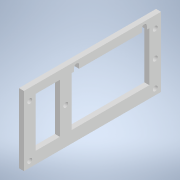
# Autodesk Inventor part: Soporte_PCB
Saved by Autodesk Inventor 2020.1 (Build 241239000, 239)
## iProperties
Created: 2019-12-12
Part Number: Soporte_PCB
Material: Generic
Document SubType Name: Modeling
Designer: Daniel
Density: 1 g/cm^3
Appearance: Default
Author: Daniel
Autodesk Inventor part; units mm, degrees
ref_plane "YZ Plane" through (0, 0, 0) normal (1, 0, 0) x (0, 1, 0)
ref_plane "XZ Plane" through (0, 0, 0) normal (0, 1, 0) x (-1, 0, 0)
ref_plane "XY Plane" through (0, 0, 0) normal (0, 0, 1) x (1, 0, 0)
sketch "Sketch1" plane through (0, 0, 0) normal (1, 0, 0) x (0, 1, 0)
  line L0 (-15.5, 37.5) -> (15.5, 37.5) construction
  line L1 (15.5, 37.5) -> (15.5, -37.5) construction
  line L2 (15.5, -37.5) -> (-15.5, -37.5) construction
  line L3 (-15.5, -37.5) -> (-15.5, 37.5) construction
  line L4 (-15.5, 37.5) -> (15.5, -37.5) construction
  line L5 (15.5, 37.5) -> (-15.5, -37.5) construction
  line L6 (-19, 41) -> (22.5, 41)
  line L7 (22.5, 41) -> (22.5, -41)
  line L8 (22.5, -41) -> (-19, -41)
  line L9 (-19, -41) -> (-19, 41)
  line L10 (-19, 41) -> (22.5, -41) construction
  line L11 (22.5, 41) -> (-19, -41) construction
  line L12 (-12, 34) -> (17.5, 34)
  line L13 (17.5, 34) -> (17.5, -34)
  line L14 (17.5, -34) -> (-12, -34)
  line L15 (-12, -34) -> (-12, 34)
  line L16 (-12, 34) -> (17.5, -34) construction
  line L17 (17.5, 34) -> (-12, -34) construction
  line L18 (-46.909, 0) -> (32.0039, 0) construction
  arc A0 (19.5, -32.5) -> (19.5, -29.5) centre (19.5, -31) ccw
  line L19 (19.5, -32.5) -> (17.5, -32.5)
  line L20 (19.5, -29.5) -> (17.5, -29.5)
  line L21 (19.5, -31) -> (19.5, -32.5) construction
  line L22 (19.5, -31) -> (19.5, -29.5) construction
  arc A1 (19.5, 8) -> (19.5, 11) centre (19.5, 9.5) ccw
  line L23 (19.5, 8) -> (17.5, 8)
  line L24 (19.5, 11) -> (17.5, 11)
  line L25 (19.5, 9.5) -> (19.5, -31) construction
  line L26 (22.5, -10.75) -> (19.5, -10.75) construction
  line L27 (17.5, 12.5) -> (-12, 12.5)
  line L28 (17.5, 19.5) -> (-12, 19.5)
  line L29 (17.5, 16) -> (-12, 16) construction
  point P0 (0, 0)
  point P1 (0, 0)
  point P2 (2.75, 0)
  point P3 (1.75, 0)
  point P4 (0, -37.5)
  point P5 (2.75, 16)
  dimension "d0" = 31
  dimension "d1" = 75
  dimension "d3" = 82
  dimension "d5" = 68
  dimension "d6" = 5
  dimension "d7" = 3.5
  dimension "d8" = 3.5
  dimension "d10" = 17.5
  dimension "d11" = 3
  dimension "d12" = 6.5
  dimension "d13" = 4
  dimension "d16" = 40.5
  dimension "d21" = 7
  dimension "d22" = 3.5
  constraints: 60 end point, 9 midpoint, 8 parallel, 8 point on line, 6 horizontal, 5 perpendicular, 4 coincident, 4 point on circle, 4 vertical, 2 centre point, 2 symmetric about line, 10 other
  measures "d0" distance of L1.end L2.end
  measures "d1" distance of L0.end L1.end
  measures "d3" distance of L6.end L7.end
  measures "d5" distance of L12.end L13.end
  measures "d6" distance between parallel lines of L7 L13
  measures "d7" distance between parallel lines of L9 L3
  measures "d8" distance between parallel lines of L15 L3
  measures "d10" distance from line of point (0, 0) L13
  measures "d11" diameter of A0
  measures "d12" distance from line of L2 L21.start
  measures "d13" distance from line of L21.start L1
  measures "d16" distance of L21.start L25.start
  measures "d21" distance between parallel lines of L27 L28
  measures "d22" distance between parallel lines of L27 L29
extrude "Extrusion1" add sketch "Sketch1" along normal blind 3 contours L6 L7 L8 L9 | L28 L13 L27 L15
hole "Hole1" at (0, 2.75, 0) at (0, 1.75, 0) at (0, 15.5, 37.5) at (0, -15.5, 37.5) at (0, -15.5, -37.5) at (0, 0, -37.5) at (0, 15.5, -37.5) at (0, 2.75, 16) direction (1, 0, 0) diameter 2.9 depth 10 tip angle 118
body "Solid1"
